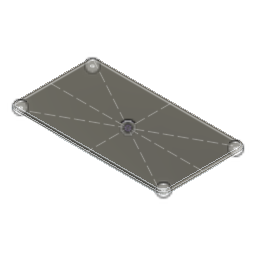
Adafruit_Solar_Panel_6V_3.5W_P500B (Autodesk Fusion 360 design; units mm, degrees)
Autodesk Fusion 360 part; units mm, degrees
sketch "Sketch1" plane through (0, 0, 0) normal (0, 0, 1) x (1, 0, 0)
  line L0 (105, 57.5) -> (-105, 57.5)
  line L1 (-105, 57.5) -> (-105, -57.5)
  line L2 (-105, -57.5) -> (105, -57.5)
  line L3 (105, -57.5) -> (105, 57.5)
  line L4 (105, 57.5) -> (-105, -57.5) construction
  line L5 (-105, 57.5) -> (105, -57.5) construction
  circle A0 centre (97.5, -49) radius 1.5
  line L6 (0, 57.5) -> (0, -57.5) construction
  line L7 (-105, 0) -> (105, 0) construction
  circle A1 centre (97.5, 49) radius 1.5
  circle A2 centre (-97.5, -49) radius 1.5
  circle A3 centre (-97.5, 49) radius 1.5
  dimension "d1" = 210
  dimension "d2" = 115
  dimension "d3" = 3
  dimension "d4" = 97.5
  dimension "d5" = 49
  constraint horizontal L0
  constraint perpendicular L0 L1
  constraint parallel L0 L2
  constraint parallel L1 L3
  constraint coincident L4 origin
  constraint coincident L5 origin
  constraint midpoint L0 L6.start
  constraint midpoint L2 L6.end
  constraint midpoint L1 L7.start
  constraint midpoint L3 L7.end
  constraint equal A0 A1
  constraint symmetric A0.centre L7 A1.centre
  constraint equal A0 A2
  constraint symmetric A0.centre L6 A2.centre
  constraint equal A2 A3
  constraint symmetric L7 A2 A3
  measures "d1" distance of L1.end L2.end
  measures "d2" distance of L0.end L1.end
  measures "d3" diameter of A0
  measures "d4" distance of A0.centre L6
  measures "d5" distance of A0.centre L7
extrude "Extrude1" add sketch "Sketch1" along normal blind 5 contours L0 L1 L2 L3 | A0 | A1 | A2 | A3
extrude "Extrude2" add sketch "Sketch1" against normal blind 5 contours A0 | A1 | A2 | A3
fillet "Fillet1" radius 10 4 edges at (-105, -57.5, 2.5) (-105, 57.5, 2.5) (105, -57.5, 2.5) (105, 57.5, 2.5)
fillet "Fillet2" radius 2 8 edges at (102.0711, -54.5711, 5) (105, 0, 5) (102.0711, 54.5711, 5) (0, 57.5, 5) (-102.0711, 54.5711, 5) (-105, 0, 5) (-102.0711, -54.5711, 5) (0, -57.5, 5)
equation "d4 = ( 195 / 2 ) * 1 mm"
equation "d5 = ( 98 / 2 ) * 1 mm"
